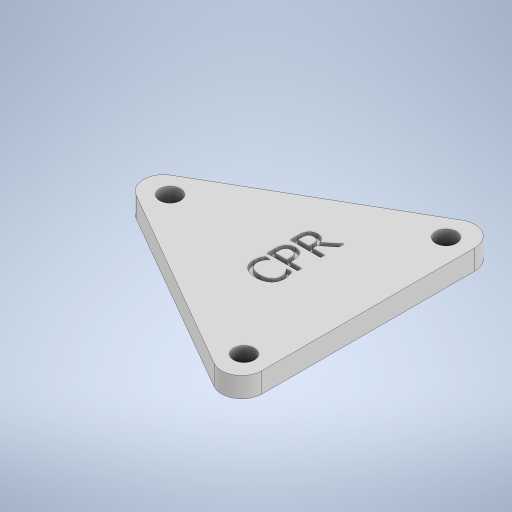
# Autodesk Inventor part: push_plate
Saved by Autodesk Inventor 2023 (Build 270158000, 158)
## iProperties
Created: 2022-11-10
Part Number: push_plate
Material: Generic
Document SubType Name: Modeling
Designer: eahil
Density: 1 g/cm^3
Appearance: Default
Author: eahil
Autodesk Inventor part; units mm, degrees
note: some values were not read from the file. Chosen so that the rebuilt part matches the saved one: direction of "Emboss1".
ref_plane "YZ Plane" through (0, 0, 0) normal (1, 0, 0) x (0, 1, 0)
ref_plane "XZ Plane" through (0, 0, 0) normal (0, 1, 0) x (-1, 0, 0)
ref_plane "XY Plane" through (0, 0, 0) normal (0, 0, 1) x (1, 0, 0)
sketch "Sketch1" plane through (0, 0, 0) normal (0, 1, 0) x (-1, 0, 0)
  circle A0 centre (0, 0) radius 5.127
  circle A1 centre (0, -100) radius 5.127
  circle A2 centre (86.6025, -50) radius 5.127
  line L0 (0, -100) -> (0, 0)
  line L1 (0, 0) -> (86.6025, -50)
  line L2 (86.6025, -50) -> (0, -100)
  line L3 (-11.547, -102.6795) -> (-11.547, 2.6795)
  line L4 (3.453, 11.3397) -> (94.6966, -41.3397)
  line L5 (94.6966, -58.6603) -> (3.453, -111.3397)
  arc A3 (94.6966, -58.6603) -> (94.6966, -41.3397) centre (89.6966, -50) ccw
  arc A4 (-11.547, -102.6795) -> (3.453, -111.3397) centre (-1.547, -102.6795) ccw
  arc A5 (3.453, 11.3397) -> (-11.547, 2.6795) centre (-1.547, 2.6795) ccw
  point P0 (28.8675, -50)
  point P1 (28.8675, -50)
  point P2 (-11.547, -120)
  point P3 (-11.547, 20)
  point P4 (109.6966, -50)
  dimension "d0" = 10.254
  dimension "d1" = 100
  dimension "d2" = 140
  dimension "d3" = 10
  constraints: 12 end point, 6 centre point, 6 point on circle, 6 point on line, 6 tangent, 5 coincident, 4 equal radius, 1 parallel, 1 vertical alignment, 14 other
  measures "d0" diameter of A0
  measures "d1" distance of A1.centre point (0, 0)
  measures "d2" distance of point (109.697, -50) point (-11.547, -120)
  measures "d3" radius of A3
extrude "Extrusion1" add sketch "Sketch1" along normal blind 10 contours A0 L1 A2 L2 A1 L0 | L3 A5 L4 A3 L5 A4
sketch "Sketch2" plane through (0, 10, 0) normal (0, 1, 0) x (1, 0, 0)
  line L0 (-37.7356, 35.0073) -> (-37.7356, 129.948) construction
  line L1 (-37.7356, 129.948) -> (141.997, 129.948) construction
  line L2 (141.997, 129.948) -> (141.997, 35.0073) construction
  line L3 (141.997, 35.0073) -> (-37.7356, 35.0073) construction
  spline S0 degree 2 poles (-22.2008, 42.3857) (-22.2008, 40.9271) (-23.1854, 38.4595) (-24.17, 37.56) knots 0 0 0 1 2 2 2
  spline S1 degree 2 poles (-24.17, 37.56) (-25.1424, 36.6605) (-28.0598, 35.6759) (-29.956, 35.6759) knots 0 0 0 1 2 2 2
  spline S2 degree 2 poles (-29.956, 35.6759) (-31.8401, 35.6759) (-34.6359, 36.6361) (-35.6692, 37.5478) knots 0 0 0 1 2 2 2
  spline S3 degree 2 poles (-35.6692, 37.5478) (-36.6781, 38.4473) (-37.7356, 40.9028) (-37.7356, 42.4222) knots 0 0 0 1 2 2 2
  spline S4 degree 2 poles (-37.7356, 42.4222) (-37.7356, 43.1759) (-37.5168, 44.5008) (-37.3466, 45.06) knots 0 0 0 1 2 2 2
  spline S5 degree 2 poles (-37.3466, 45.06) (-37.1886, 45.5462) (-36.7388, 46.5551) (-36.4714, 47.0535) knots 0 0 0 1 2 2 2
  line L4 (-36.4714, 47.0535) -> (-34.0646, 47.0535)
  line L5 (-34.0646, 47.0535) -> (-34.0646, 46.8955)
  spline S6 degree 2 poles (-34.0646, 46.8955) (-34.3077, 46.628) (-34.9884, 45.8015) (-35.3166, 45.2058) knots 0 0 0 1 2 2 2
  spline S7 degree 2 poles (-35.3166, 45.2058) (-35.6327, 44.6345) (-36.0338, 43.2853) (-36.0338, 42.4101) knots 0 0 0 1 2 2 2
  spline S8 degree 2 poles (-36.0338, 42.4101) (-36.0338, 41.4498) (-35.2437, 39.7358) (-34.4901, 39.0916) knots 0 0 0 1 2 2 2
  spline S9 degree 2 poles (-34.4901, 39.0916) (-33.7243, 38.4595) (-31.4025, 37.7545) (-29.956, 37.7545) knots 0 0 0 1 2 2 2
  spline S10 degree 2 poles (-29.956, 37.7545) (-28.4123, 37.7545) (-26.1878, 38.4959) (-25.422, 39.1402) knots 0 0 0 1 2 2 2
  spline S11 degree 2 poles (-25.422, 39.1402) (-24.6805, 39.7723) (-23.9269, 41.4619) (-23.9269, 42.4101) knots 0 0 0 1 2 2 2
  spline S12 degree 2 poles (-23.9269, 42.4101) (-23.9269, 43.2731) (-24.3523, 44.7439) (-24.6683, 45.3152) knots 0 0 0 1 2 2 2
  spline S13 degree 2 poles (-24.6683, 45.3152) (-24.9844, 45.8622) (-25.6408, 46.6767) (-25.8717, 46.9076) knots 0 0 0 1 2 2 2
  line L6 (-25.8717, 46.9076) -> (-25.8717, 47.0535)
  line L7 (-25.8717, 47.0535) -> (-23.4893, 47.0535)
  spline S14 degree 2 poles (-23.4893, 47.0535) (-23.2583, 46.5551) (-22.8329, 45.6799) (-22.6384, 45.06) knots 0 0 0 1 2 2 2
  spline S15 degree 2 poles (-22.6384, 45.06) (-22.4196, 44.4036) (-22.2008, 43.2853) (-22.2008, 42.3857) knots 0 0 0 1 2 2 2
  spline S16 degree 2 poles (-32.9463, 58.3947) (-31.9739, 58.3947) (-30.2234, 57.7018) (-29.6157, 57.0818) knots 0 0 0 1 2 2 2
  spline S17 degree 2 poles (-29.6157, 57.0818) (-28.8499, 56.3039) (-28.0598, 54.201) (-28.0598, 52.5964) knots 0 0 0 1 2 2 2
  line L8 (-28.0598, 52.5964) -> (-28.0598, 50.9068)
  line L9 (-28.0598, 50.9068) -> (-22.4682, 50.9068)
  line L10 (-22.4682, 50.9068) -> (-22.4682, 48.9133)
  line L11 (-22.4682, 48.9133) -> (-37.4682, 48.9133)
  line L12 (-37.4682, 48.9133) -> (-37.4682, 52.6815)
  spline S18 degree 2 poles (-37.4682, 52.6815) (-37.4682, 54.0186) (-37.0306, 55.8906) (-36.5322, 56.6078) knots 0 0 0 1 2 2 2
  spline S19 degree 2 poles (-36.5322, 56.6078) (-35.9609, 57.4465) (-34.1983, 58.3947) (-32.9463, 58.3947) knots 0 0 0 1 2 2 2
  spline S20 degree 2 poles (-32.8855, 56.316) (-33.6635, 56.316) (-34.8061, 55.7812) (-35.1708, 55.2342) knots 0 0 0 1 2 2 2
  spline S21 degree 2 poles (-35.1708, 55.2342) (-35.4868, 54.7601) (-35.7421, 53.4959) (-35.7421, 52.56) knots 0 0 0 1 2 2 2
  line L13 (-35.7421, 52.56) -> (-35.7421, 50.9068)
  line L14 (-35.7421, 50.9068) -> (-29.7615, 50.9068)
  line L15 (-29.7615, 50.9068) -> (-29.7615, 52.2682)
  spline S22 degree 2 poles (-29.7615, 52.2682) (-29.7615, 53.4838) (-30.1505, 54.9789) (-30.6611, 55.4652) knots 0 0 0 1 2 2 2
  spline S23 degree 2 poles (-30.6611, 55.4652) (-31.1108, 55.9149) (-32.1683, 56.316) (-32.8855, 56.316) knots 0 0 0 1 2 2 2
  line L16 (-22.4682, 71.8995) -> (-22.4682, 69.3104)
  line L17 (-22.4682, 69.3104) -> (-28.4366, 64.5697)
  line L18 (-28.4366, 64.5697) -> (-28.4366, 62.2844)
  line L19 (-28.4366, 62.2844) -> (-22.4682, 62.2844)
  line L20 (-22.4682, 62.2844) -> (-22.4682, 60.2909)
  line L21 (-22.4682, 60.2909) -> (-37.4682, 60.2909)
  line L22 (-37.4682, 60.2909) -> (-37.4682, 64.1564)
  spline S24 degree 2 poles (-37.4682, 64.1564) (-37.4682, 65.4449) (-37.1886, 67.1831) (-36.6781, 67.9733) knots 0 0 0 1 2 2 2
  spline S25 degree 2 poles (-36.6781, 67.9733) (-36.1675, 68.7634) (-34.5752, 69.675) (-33.3961, 69.675) knots 0 0 0 1 2 2 2
  spline S26 degree 2 poles (-33.3961, 69.675) (-31.7551, 69.675) (-29.5306, 67.9976) (-28.9957, 66.5632) knots 0 0 0 1 2 2 2
  line L23 (-28.9957, 66.5632) -> (-22.4682, 71.8995)
  spline S27 degree 2 poles (-33.238, 67.5964) (-33.8944, 67.5964) (-34.9034, 67.1345) (-35.2316, 66.6483) knots 0 0 0 1 2 2 2
  spline S28 degree 2 poles (-35.2316, 66.6483) (-35.5111, 66.2229) (-35.7421, 65.0924) (-35.7421, 64.2658) knots 0 0 0 1 2 2 2
  line L24 (-35.7421, 64.2658) -> (-35.7421, 62.2844)
  line L25 (-35.7421, 62.2844) -> (-30.1019, 62.2844)
  line L26 (-30.1019, 62.2844) -> (-30.1019, 64.0348)
  spline S29 degree 2 poles (-30.1019, 64.0348) (-30.1019, 64.8979) (-30.4058, 66.2715) (-30.8799, 66.7455) knots 0 0 0 1 2 2 2
  spline S30 degree 2 poles (-30.8799, 66.7455) (-31.2931, 67.1831) (-32.4601, 67.5964) (-33.238, 67.5964) knots 0 0 0 1 2 2 2
  point P0 (0, 0)
  constraints: 2 other
emboss "Emboss1" sketch "Sketch2" operation cut depth 2 direction (0, -1, 0)
body "Solid1"
